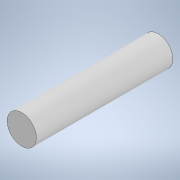
# Autodesk Inventor part: 棒
Saved by Autodesk Inventor 2022 (Build 260153070, 153G)
## iProperties
Created: 2022-09-26
Part Number: 棒
Material: 一般
Document SubType Name: Modeling
Designer: hirok
Density: 1 g/cm^3
Appearance: 既定
Author: hirok
Autodesk Inventor part; units mm, degrees
ref_plane "YZ Plane" through (0, 0, 0) normal (1, 0, 0) x (0, 1, 0)
ref_plane "XZ Plane" through (0, 0, 0) normal (0, 1, 0) x (-1, 0, 0)
ref_plane "XY Plane" through (0, 0, 0) normal (0, 0, 1) x (1, 0, 0)
sketch "スケッチ1" plane through (0, 0, 0) normal (0, 0, 1) x (1, 0, 0)
  circle A0 centre (0, 0) radius 1.5
  dimension "d0" = 3
  constraints: 1 centre point, 1 coincident
  measures "d0" diameter of A0
extrude "押し出し1" add sketch "スケッチ1" along normal blind 14
